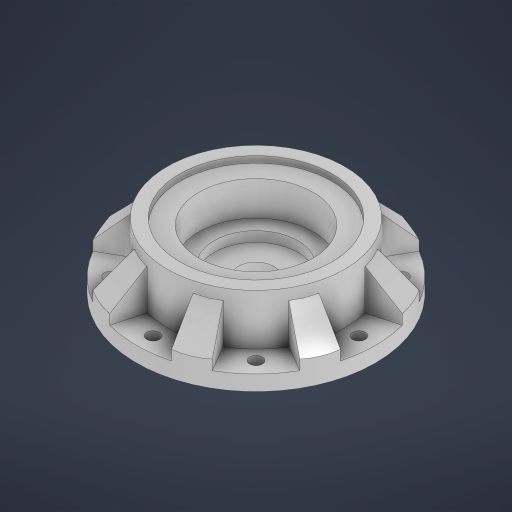
# Autodesk Inventor part: A_axisShesterna
Saved by Autodesk Inventor 2024 (Build 280153000, 153)
## iProperties
Created: 2023-12-22
Part Number: A_axisShesterna
Material: Aluminum 6061-AHC
Document SubType Name: Modeling
Designer: KirikDK
Mass: 2040.33 g
Surface Area: 991.497 cm^2
Volume: 755.678 cm^3
Density: 2.7 g/cm^3
Appearance: Aluminum - Dark
Author: KirikDK
Autodesk Inventor part; units mm, degrees
ref_plane "YZ Plane" through (0, 0, 0) normal (1, 0, 0) x (0, 1, 0)
ref_plane "XZ Plane" through (0, 0, 0) normal (0, 1, 0) x (-1, 0, 0)
ref_plane "XY Plane" through (0, 0, 0) normal (0, 0, 1) x (1, 0, 0)
sketch "Sketch1" plane through (0, 0, 0) normal (0, 1, 0) x (-1, 0, 0)
  circle A0 centre (0, 0) radius 125
  dimension "d0" = 250
  constraints: 1 centre point, 1 coincident
  measures "d0" diameter of A0
extrude "Extrusion1" add sketch "Sketch1" along normal blind 12
sketch "Sketch2" plane through (0, 12, 0) normal (0, 1, 0) x (1, 0, 0)
  circle A0 centre (0, 0) radius 125 projected
  circle A1 centre (0, 0) radius 70
  circle A2 centre (0, 0) radius 45
  dimension "d10" = 90
  dimension "d11" = 140
  constraints: 2 centre point, 2 coincident
  measures "d10" diameter of A2
  measures "d11" diameter of A1
extrude "Extrusion2" add sketch "Sketch2" along normal blind 40 contours A1
sketch "Sketch3" plane through (0, 12, 0) normal (0, 1, 0) x (1, 0, 0)
  circle A0 centre (0, -124.7208) radius 1.2635
  point P0 (0, 0)
  constraints: 1 centre point
extrude "Extrusion3" cut sketch "Sketch3" against normal blind 10
pattern_circular "Circular Pattern1" count 180 over 360 about axis through (0, 12, 0) along (0, 1, 0) of "Extrusion3"
sketch "Sketch4" plane through (0, 12, 0) normal (0, 1, 0) x (1, 0, 0)
  circle A0 centre (0, 0) radius 45 projected
  circle A1 centre (0, 0) radius 33
  constraints: 1 centre point, 1 coincident
extrude "Extrusion4" add sketch "Sketch4" along normal blind 8
sketch "Sketch5" plane through (0, 52, 0) normal (0, 1, 0) x (1, 0, 0)
  circle A0 centre (0, 0) radius 60
  constraints: 1 centre point, 1 coincident
extrude "Extrusion5" cut sketch "Sketch5" against normal blind 5
sketch "Sketch6" plane through (0, 12, 0) normal (0, 1, 0) x (1, 0, 0)
  circle A0 centre (0, 0) radius 14
  constraints: 1 centre point, 1 coincident
extrude "Extrusion6" cut sketch "Sketch6" against normal blind 25
sketch "Sketch7" plane through (0, 12, 0) normal (0, 1, 0) x (1, 0, 0)
  circle A0 centre (-81, 0) radius 5
  circle A1 centre (-57.2756, -57.2756) radius 5
  circle A2 centre (0, -81) radius 5
  circle A3 centre (57.2756, -57.2756) radius 5
  circle A4 centre (81, 0) radius 5
  circle A5 centre (57.2756, 57.2756) radius 5
  circle A6 centre (0, 81) radius 5
  circle A7 centre (-57.2756, 57.2756) radius 5
  point P0 (0, 0)
  dimension "d20" = 360
  constraints: 8 centre point, 17 other
extrude "Extrusion7" cut sketch "Sketch7" against normal blind 20
sketch "Sketch8" plane through (0, 12, 0) normal (0, 1, 0) x (1, 0, 0)
  line L0 (0, 0) -> (-120.7407, 32.3524)
  circle A0 centre (0, 0) radius 125 projected
  line L1 (0, 0) -> (-108.2532, 62.5)
  line L2 (0, 0) -> (-127, 0)
  line L3 (-127, 0) -> (-127, 138)
  line L4 (-127, 138) -> (0, 138)
  line L5 (0, 138) -> (0, 0)
  line L6 (0, 0) -> (-82.0122, 33.9706)
  line L7 (-102.4786, 16.8742) -> (-85.0906, 58.8526)
  circle A1 centre (0, 0) radius 70
  point P0 (-67.6148, 18.1173)
  point P1 (-60.6218, 35)
  point P2 (-88.3416, 51.004)
  point P3 (-98.5322, 26.4016)
  dimension "d24" = 15
  dimension "d25" = 60
  dimension "d26" = 7.5
  dimension "d27" = 7.5
  constraints: 16 end point, 2 parallel, 2 perpendicular, 2 point on circle, 1 centre point, 1 coincident, 1 horizontal
  measures "d24" angle of L2 L0
  measures "d25" angle of L5 L1
  measures "d26" angle of L1 L6
  measures "d27" angle of L0 L6
extrude "Extrusion8" add sketch "Sketch8" along normal blind 31.5 contours L0 L7 L1 A1
chamfer "Chamfer1" distance 31.5 angle 45 1 edges at (-93.4369, 43.5, -38.7028)
pattern_circular "Circular Pattern2" count 8 over 360 about axis through (0, 12, 0) along (0, 1, 0) of "Extrusion8", "Chamfer1"
sketch "Sketch10" plane through (0, 12, 0) normal (0, 1, 0) x (1, 0, 0)
  circle A0 centre (0, 0) radius 94
  circle A1 centre (0, 0) radius 128
  constraints: 2 centre point, 2 coincident
extrude "Extrusion10" cut sketch "Sketch10" along normal mid plane 100
body "Solid1"
